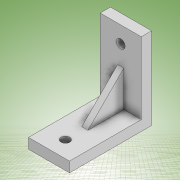
# Autodesk Inventor part: Escuadra
Saved by Autodesk Inventor 2022 (Build 260153000, 153)
## iProperties
Created: 2022-03-11
Part Number: Escuadra
Material: Genérico
Document SubType Name: Modeling
Designer: Marco
Density: 1 g/cm^3
Appearance: Valor por defecto
Author: Marco
Autodesk Inventor part; units mm, degrees
ref_plane "YZ Plane" through (0, 0, 0) normal (1, 0, 0) x (0, 1, 0)
ref_plane "XZ Plane" through (0, 0, 0) normal (0, 1, 0) x (-1, 0, 0)
ref_plane "XY Plane" through (0, 0, 0) normal (0, 0, 1) x (1, 0, 0)
sketch "Boceto1" plane through (0, 0, 0) normal (0, 0, 1) x (1, 0, 0)
  line L0 (0, 0) -> (20, 0)
  line L1 (20, 0) -> (20, 40)
  line L2 (20, 40) -> (0, 40)
  line L3 (0, 40) -> (0, 0)
  circle A0 centre (10, 32) radius 2.15
  point P0 (10, 40)
  dimension "d0" = 20
  dimension "d1" = 40
  dimension "d14" = 4.3
  dimension "d15" = 8
  constraints: 8 end point, 2 parallel, 1 centre point, 1 horizontal, 1 midpoint, 1 perpendicular, 1 vertical alignment
  measures "d0" distance of L2.end L1.end
  measures "d1" distance of L1.end L0.end
  measures "d14" diameter of A0
  measures "d15" vertical distance of A0.centre L2.end
extrude "Extrusión1" add sketch "Boceto1" along normal blind 5
sketch "Boceto2" plane through (0, 0, 5) normal (0, 0, 1) x (1, 0, 0)
  line L0 (20, 0) -> (20, 40) projected
  line L1 (0, 0) -> (20, 0)
  line L2 (20, 0) -> (20, 5)
  line L3 (20, 5) -> (0, 5)
  line L4 (0, 5) -> (0, 0)
  dimension "d4" = 5
  constraints: 8 end point, 2 parallel, 1 horizontal, 1 perpendicular, 1 point on line
  measures "d4" distance of L1.start L3.end
extrude "Extrusión2" add sketch "Boceto2" along normal blind 35
ref_plane "Plano de trabajo1" through (10, 0, 0) normal (1, 0, 0) x (0, 0, -1)
sketch "Boceto3" plane through (10, 0, 0) normal (1, 0, 0) x (0, 0, -1)
  line L0 (-5, 5) -> (-5, 40) projected
  line L1 (-5, 5) -> (-40, 5) projected
  line L2 (-22.5, 5) -> (-5, 22.5)
  line L3 (-5, 40) -> (-5, 5) projected
  point P0 (0, 0)
  dimension "d7" = 45
  constraints: 2 end point, 2 midpoint
  measures "d7" angle of L1 L2
extrude "Nervio1" add sketch "Boceto3" along normal mid plane 3 rib yes fills toward (-13.7146, 13.7146) open curves L2
sketch "Boceto4" plane through (0, 5, 40) normal (0, 1, 0) x (1, 0, 0)
  line L0 (20, 0) -> (0, 0) projected
  circle A0 centre (10, 8) radius 2.15
  point P0 (0, 40)
  point P1 (10, 0)
  dimension "d16" = 4.3
  dimension "d17" = 8
  constraints: 1 centre point, 1 midpoint, 1 vertical alignment
  measures "d16" diameter of A0
  measures "d17" vertical distance of L0.start A0.centre
extrude "Extrusión3" cut sketch "Boceto4" against normal up to surface (5 mm away)
